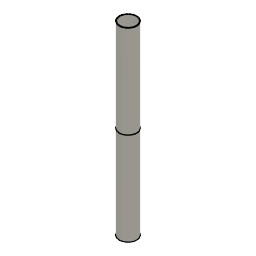
Upper and Lower Body Tube (Autodesk Fusion 360 design; units mm, degrees)
part number: 2026-02-28-23-49-06-341
part number: 2026-02-28-23-54-10-794
Autodesk Fusion 360 part; units mm, degrees
sketch "Sketch1" plane through (0, 0, 0) normal (0, 1, 0) x (1, 0, 0)
  circle A0 centre (0, 0) radius 33
  circle A1 centre (0, 0) radius 31
  dimension "d1" = 66
  dimension "d2" = 62
  constraint coincident A0.centre A1.centre
  measures "d1" diameter of A0
  measures "d2" diameter of A1
extrude "Extrude1" add sketch "Sketch1" along normal blind 350 makes body 1
ref_plane "WorkPlane1" through (0, 350, 0) normal (0, 1, 0) x (1, 0, 0)
sketch "Sketch2" plane through (0, 350, 0) normal (0, 1, 0) x (1, 0, 0)
  circle A0 centre (0, 0) radius 31
  circle A1 centre (0, 0) radius 33
extrude "Extrude1'" add sketch "Sketch2" along normal blind 350 separate body makes body 2 in component "Upper Body Tube"
component "Upper Body Tube" placed x (1, 0, 0) y (0, 1, 0) z (0, 0, 1) at (0, 0, 0)
named bodies: "Lower Body Tube"
